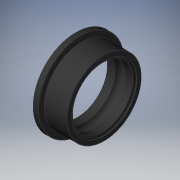
# Autodesk Inventor part: SKF_W 624 R_PART2
Saved by Autodesk Inventor 2019 (Build 230136000, 136)
## iProperties
Created: 2022-09-09
Part Number: SKF_W 624 R_PART2
Material: Generic
Catalog Web Link: www.cadenas.de
Description: -Deep groove ball bearings
Vendor: SKF
Document SubType Name: Modeling
Designer: psAdmin
Manufacturer: SKF
Mass: 3 g
Surface Area: 5.55762 cm^2
Volume: 0.258277 cm^3
Density: 1 g/cm^3
Appearance: PSOLRGB-175-175-175
Category: PARTsolutions
Company: SKF
Title: SKF_W 624 R_PART2
Author: Cadenas PARTsolutions
Comments: Deep groove ball bearings
PSOL_IDENT_0: {$CADENAS_DATA/23d-libs/skf/bearings_units_and_housings/ball_bearings/deep_groove_ball_bearings/bb1_
PSOL_IDENT_1: 001_101.prj},201 {VTYP=3D},{NB=SKF_W 624 R_PART2},{LINA=SKF_W 624 R_PART2},{NN=BB1_001_101_PART2},{N
PSOL_IDENT_2: OPRJ=TRUE},{DATE=04.08.2022 15:25:15},{GEOMDATE=04.07.2022 10:54:51},{VERSION=},{LINEID=21510},{WBVA
PSOL_IDENT_3: R=},{WBNUMERIC=}  {NB=SKF_W 624 R_PART2},{LINA=SKF_W 624 R_PART2},{KT=DUMMY},{DESIGNATION=W 624 R},{
PSOL_IDENT_4: R12=0.20},{DD=4.000},{D=13.000},{B=5.000},{C=},{CX=},{CXX=1},{CA=1.000},{XXVARIANT=Flanged outer rin
PSOL_IDENT_5: g},{XXDESIGN=Single row stainless steel},{XXSEALING=No seals},{DESIGN=dgbbwr2zs},{DESIGNIR=dgbbwr2zs
PSOL_IDENT_6: },{VARIANT=Flanged outer ring},{DD1=6.95},{DD2=6},{DD2X=},{DD2A=6.00},{D1=10.45},{D1X=0.00},{D2=11.3
PSOL_IDENT_7: 5},{D2A=11.35},{D3=15},{D3X=},{D3A=15.000},{D4=},{HH=0.000},{BB=0.000},{BBX=},{BBA=0.000},{FF=},{R0M
PSOL_IDENT_8: AX=0.000},{R0=0.000},{PITCH=8.70},{DW=2.381},{DDAMIN=5.600},{DDAMAX=0.000},{DDBMIN=0.000},{DDBMAX=0.
PSOL_IDENT_9: 000},{DBMIN=0.000},{DAMAX=0.000},{BBAMIN=0.000},{CAMAX=0.000},{RAMAX=0.200},{LOAD1=0.741},{LOAD2=0.2
PSOL_IDENT_10: 50},{LOAD3=0.011},{SPEED1=110000},{SPEED2=70000},{KR=0.030},{F0=6.400},{Z=7},{II=1},{MASS=0.003},{BE
PSOL_IDENT_11: ARING=W 624 R},{RING=},{HELP=1.275},{HELP2=0.825},{DD1ALG=3.475},{YALG=3.475},{PITCH1=8.700},{DW1=2.
PSOL_IDENT_12: 381},{YALG1=5.225},{HALG1=1.275},{SH=3.000},{CU=0.524},{HALG=1.475},{B1=-2.82145},{SHIELDHELP=1},{D4
PSOL_IDENT_13: A=0.000},{FFA=0.000},{RS1=},{HELP3=0}
NB: SKF_W 624 R_PART2
NT: Deep groove ball bearings
NBSYN: SKF_$DESIGNATION._PART2
LINA: SKF_W 624 R_PART2
CATALOG: SKF
DESIGNATION: W 624 R
R12: 0.2
DD: 4
D: 13
B: 5
XXVARIANT: Flanged outer ring
XXDESIGN: Single row stainless steel
XXSEALING: No seals
DD2: 6
D2: 11.35
LOAD1: 0.741
LOAD2: 0.25
LOAD3: 0.011
SPEED1: 110000
SPEED2: 70000
BEARING: W 624 R
SUPPLIER: SKF
ARTICLENO: SKF_W 624 R_PART2
BOMINFO: SKF_W 624 R_PART2
CREATOR: CADENAS GmbH
Autodesk Inventor part; units mm, degrees
ref_plane "YZ Plane" through (0, 0, 0) normal (1, 0, 0) x (0, 1, 0)
ref_plane "XZ Plane" through (0, 0, 0) normal (0, 1, 0) x (-1, 0, 0)
ref_plane "XY Plane" through (0, 0, 0) normal (0, 0, 1) x (1, 0, 0)
sketch "Sketch_21" plane through (0, 0, 0) normal (0, 0, 1) x (1, 0, 0)
  line L0 (50, 0) -> (-50, 0)
  line L1 (0, 7.4333) -> (0, 5.675)
  line L2 (0, 5.675) -> (0.1, 5.675)
  arc A0 (0.3, 5.475) -> (0.1, 5.675) centre (0.1, 5.475) ccw
  line L3 (0.3, 5.475) -> (0.3, 5.225)
  line L4 (0.3, 5.225) -> (1.6927, 5.225)
  arc A1 (3.3073, 5.225) -> (1.6927, 5.225) centre (2.5, 4.35) ccw
  line L5 (3.3073, 5.225) -> (4.7, 5.225)
  line L6 (4.7, 5.225) -> (4.7, 5.475)
  arc A2 (4.9, 5.675) -> (4.7, 5.475) centre (4.9, 5.475) ccw
  line L7 (4.9, 5.675) -> (5, 5.675)
  line L8 (5, 5.675) -> (5, 6.4333)
  arc A3 (5, 6.4333) -> (4.9333, 6.5) centre (4.9333, 6.4333) ccw
  line L9 (4.9333, 6.5) -> (1, 6.5)
  line L10 (1, 6.5) -> (1, 7.4333)
  arc A4 (1, 7.4333) -> (0.9333, 7.5) centre (0.9333, 7.4333) ccw
  line L11 (0.9333, 7.5) -> (0.0667, 7.5)
  arc A5 (0.0667, 7.5) -> (0, 7.4333) centre (0.0667, 7.4333) ccw
  constraints: 24 end point, 12 point on circle, 6 centre point
revolve "Revolution1" add sketch "Sketch_21" angle 360 about axis through (50, 0, 0) along (1, 0, 0)
body "Solid1"
